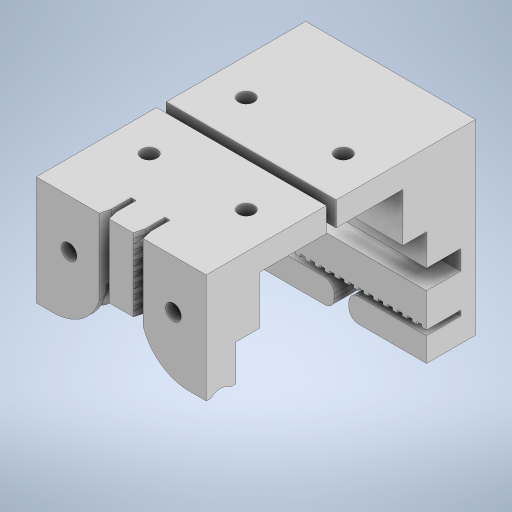
# Autodesk Inventor part: carriage
Saved by Autodesk Inventor 2023.1 (Build 271208000, 208)
## iProperties
Created: 2022-11-02
Part Number: carriage
Material: Generic
Document SubType Name: Modeling
Designer: nicol
Density: 1 g/cm^3
Appearance: Default
Author: nicol
Autodesk Inventor part; units mm, degrees
ref_plane "YZ Plane" through (0, 0, 0) normal (1, 0, 0) x (0, 1, 0)
ref_plane "XZ Plane" through (0, 0, 0) normal (0, 1, 0) x (-1, 0, 0)
ref_plane "XY Plane" through (0, 0, 0) normal (0, 0, 1) x (1, 0, 0)
sketch "Sketch1" plane through (0, 0, 0) normal (0, 1, 0) x (-1, 0, 0)
  line L0 (0, 0) -> (35, 0)
  line L1 (35, 0) -> (35, -55.5)
  line L2 (35, -55.5) -> (0, -55.5)
  line L3 (0, -55.5) -> (0, 0)
  line L4 (27.5, -15.75) -> (7.5, -15.75) construction
  line L5 (7.5, -15.75) -> (7.5, -35.75) construction
  line L6 (7.5, -35.75) -> (27.5, -35.75) construction
  line L7 (27.5, -35.75) -> (27.5, -15.75) construction
  dimension "d0" = 20
  dimension "d1" = 20
  dimension "d2" = 15.75
  dimension "d3" = 19.75
  dimension "d4" = 35
  dimension "d5" = 7.5
  dimension "d6" = 7.5
  constraints: 16 end point, 4 parallel, 2 horizontal, 2 perpendicular
  measures "d0" distance of L6.end L5.end
  measures "d1" distance of L5.end L4.end
  measures "d2" distance between parallel lines of L0 L4
  measures "d3" distance between parallel lines of L2 L6
  measures "d4" distance of L0.start L0.end
  measures "d5" distance between parallel lines of L1 L7
  measures "d6" distance between parallel lines of L3 L5
extrude "Extrusion1" add sketch "Sketch1" against normal blind 5
hole "Hole1" at (-27.5, 0, -15.75) at (-7.5, 0, -15.75) at (-27.5, 0, -35.75) at (-7.5, 0, -35.75) direction (0, -1, 0) diameter 3.2 end through all
sketch "Sketch2" plane through (0, -5, 0) normal (0, -1, 0) x (1, 0, 0)
  circle A0 centre (-27.5, -35.75) radius 1.6 projected
  circle A1 centre (-27.5, -15.75) radius 1.6 projected
  circle A2 centre (-7.5, -15.75) radius 1.6 projected
  circle A3 centre (-7.5, -35.75) radius 1.6 projected
  line L0 (-35, -55.5) -> (0, -55.5) projected
  line L1 (0, -55.5) -> (0, 0) projected
  line L2 (0, 0) -> (-35, 0) projected
  line L3 (-35, 0) -> (-35, -55.5) projected
  line L4 (0, -40.5) -> (-35, -40.5)
  line L5 (-35, -55.5) -> (-35, 0) projected
  line L6 (-35, -11) -> (0, -11)
  line L7 (0, 0) -> (0, -55.5) projected
  point P0 (0, -11)
  dimension "d16" = 11
  dimension "d17" = 15
  constraints: 4 end point, 4 point on line, 1 horizontal, 1 parallel
  measures "d16" distance between parallel lines of L2 L6
  measures "d17" distance between parallel lines of L0 L4
extrude "Extrusion2" add sketch "Sketch2" along normal blind 17.5 contours L3 L4 L1 L0 | L3 L2 L1 L6
sketch "Sketch4" plane through (-35, 0, 0) normal (0, 0, 1) x (1, 0, 0)
  line L0 (0, -22.5) -> (3.5, -22.5)
  line L1 (0, 0) -> (35, 0) projected
  line L2 (0, 0) -> (0, -22.5) projected
  line L3 (35, -22.5) -> (0, -22.5) projected
  line L4 (35, 0) -> (35, -22.5) projected
  line L5 (0, -22.5) -> (0, -26) construction
  line L6 (0, -5) -> (0, -22.5) construction
  circle A0 centre (-97.8915, -18) radius 4.5 construction
  line L7 (15, 0) -> (20, 0)
  line L8 (20, 0) -> (20, -15)
  line L9 (20, -15) -> (15, -15)
  line L10 (15, -15) -> (15, 0)
  line L11 (13.5, 0) -> (13.5, -12.5)
  arc A1 (3.5, -22.5) -> (13.5, -12.5) centre (3.5, -12.5) ccw
  line L12 (15, 0) -> (14.5, 0)
  line L13 (14.5, 0) -> (14.5, -1)
  line L14 (14.5, -1) -> (15, -1)
  line L15 (15, -1) -> (15, 0)
  line L16 (20, 0) -> (20.5, 0)
  line L17 (20.5, 0) -> (20.5, -1)
  line L18 (20.5, -1) -> (20, -1)
  line L19 (20, -1) -> (20, 0)
  line L20 (21.5, 0) -> (21.5, -12.5)
  line L21 (35, 0) -> (35, -22.5) projected
  line L22 (35, -22.5) -> (31.5, -22.5)
  arc A2 (21.5, -12.5) -> (31.5, -22.5) centre (31.5, -12.5) ccw
  line L23 (15, 0) -> (14.5, -0.5) construction
  line L24 (15, -1) -> (14.5, -0.5) construction
  line L25 (20, 0) -> (20.5, -0.5) construction
  line L26 (20, -1) -> (20.5, -0.5) construction
  line L27 (20, -3) -> (20.5, -2.5) construction
  line L28 (20, -3) -> (20, -2)
  line L29 (20, -2) -> (20.5, -2)
  line L30 (20, -2) -> (20.5, -2.5) construction
  line L31 (20.5, -3) -> (20, -3)
  line L32 (20.5, -2) -> (20.5, -3)
  line L33 (15, -2) -> (14.5, -2.5) construction
  line L34 (15, -3) -> (15, -2)
  line L35 (14.5, -3) -> (15, -3)
  line L36 (14.5, -2) -> (14.5, -3)
  line L37 (15, -2) -> (14.5, -2)
  line L38 (15, -3) -> (14.5, -2.5) construction
  line L39 (20, -5) -> (20.5, -4.5) construction
  line L40 (20, -5) -> (20, -4)
  line L41 (20, -4) -> (20.5, -4)
  line L42 (20, -4) -> (20.5, -4.5) construction
  line L43 (20.5, -5) -> (20, -5)
  line L44 (20.5, -4) -> (20.5, -5)
  line L45 (15, -4) -> (14.5, -4.5) construction
  line L46 (15, -5) -> (15, -4)
  line L47 (14.5, -5) -> (15, -5)
  line L48 (14.5, -4) -> (14.5, -5)
  line L49 (15, -4) -> (14.5, -4)
  line L50 (15, -5) -> (14.5, -4.5) construction
  line L51 (20, -7) -> (20.5, -6.5) construction
  line L52 (20, -7) -> (20, -6)
  line L53 (20, -6) -> (20.5, -6)
  line L54 (20, -6) -> (20.5, -6.5) construction
  line L55 (20.5, -7) -> (20, -7)
  line L56 (20.5, -6) -> (20.5, -7)
  line L57 (15, -6) -> (14.5, -6.5) construction
  line L58 (15, -7) -> (15, -6)
  line L59 (14.5, -7) -> (15, -7)
  line L60 (14.5, -6) -> (14.5, -7)
  line L61 (15, -6) -> (14.5, -6)
  line L62 (15, -7) -> (14.5, -6.5) construction
  line L63 (20, -9) -> (20.5, -8.5) construction
  line L64 (20, -9) -> (20, -8)
  line L65 (20, -8) -> (20.5, -8)
  line L66 (20, -8) -> (20.5, -8.5) construction
  line L67 (20.5, -9) -> (20, -9)
  line L68 (20.5, -8) -> (20.5, -9)
  line L69 (15, -8) -> (14.5, -8.5) construction
  line L70 (15, -9) -> (15, -8)
  line L71 (14.5, -9) -> (15, -9)
  line L72 (14.5, -8) -> (14.5, -9)
  line L73 (15, -8) -> (14.5, -8)
  line L74 (15, -9) -> (14.5, -8.5) construction
  line L75 (20, -11) -> (20.5, -10.5) construction
  line L76 (20, -11) -> (20, -10)
  line L77 (20, -10) -> (20.5, -10)
  line L78 (20, -10) -> (20.5, -10.5) construction
  line L79 (20.5, -11) -> (20, -11)
  line L80 (20.5, -10) -> (20.5, -11)
  line L81 (15, -10) -> (14.5, -10.5) construction
  line L82 (15, -11) -> (15, -10)
  line L83 (14.5, -11) -> (15, -11)
  line L84 (14.5, -10) -> (14.5, -11)
  line L85 (15, -10) -> (14.5, -10)
  line L86 (15, -11) -> (14.5, -10.5) construction
  line L87 (20, -13) -> (20.5, -12.5) construction
  line L88 (20, -13) -> (20, -12)
  line L89 (20, -12) -> (20.5, -12)
  line L90 (20, -12) -> (20.5, -12.5) construction
  line L91 (20.5, -13) -> (20, -13)
  line L92 (20.5, -12) -> (20.5, -13)
  line L93 (15, -12) -> (14.5, -12.5) construction
  line L94 (15, -13) -> (15, -12)
  line L95 (14.5, -13) -> (15, -13)
  line L96 (14.5, -12) -> (14.5, -13)
  line L97 (15, -12) -> (14.5, -12)
  line L98 (15, -13) -> (14.5, -12.5) construction
  line L99 (20, -15) -> (20.5, -14.5) construction
  line L100 (20, -15) -> (20, -14)
  line L101 (20, -14) -> (20.5, -14)
  line L102 (20, -14) -> (20.5, -14.5) construction
  line L103 (20.5, -15) -> (20, -15)
  line L104 (20.5, -14) -> (20.5, -15)
  line L105 (15, -14) -> (14.5, -14.5) construction
  line L106 (15, -15) -> (15, -14)
  line L107 (14.5, -15) -> (15, -15)
  line L108 (14.5, -14) -> (14.5, -15)
  line L109 (15, -14) -> (14.5, -14)
  line L110 (15, -15) -> (14.5, -14.5) construction
  point P0 (0, -24.25)
  point P1 (17.5, 0)
  point P2 (14.5, 0)
  point P3 (3.5, -22.5)
  point P4 (31.5, -22.5)
  dimension "d48" = 5
  dimension "d49" = 1.5
  dimension "d50" = 0.5
  dimension "d51" = 1
  dimension "d59" = 10
  dimension "d60" = 0.5
  dimension "d61" = 1
  dimension "d88" = 15
  dimension "d210" = 2
  constraints: 210 end point, 6 parallel, 6 point on line, 5 midpoint, 5 tangent, 4 horizontal, 4 point on circle, 3 perpendicular, 3 vertical, 2 centre point, 2 collinear, 2 equal length, 154 other
  measures "d48" distance of L8.end L9.end
  measures "d49" distance between parallel lines of L10 L11
  measures "d50" distance of L13.end L14.end
  measures "d51" distance of L12.end L13.end
  measures "d59" radius of A1
  measures "d60" distance of L17.end L18.end
  measures "d61" distance of L16.end L17.end
  measures "d88" distance between parallel lines of L1 L9
  measures "d210" distance of L18.end L27.start
extrude "Extrusion5" cut sketch "Sketch4" against normal blind 6 contours A1 L11 L1 L13 L14 L10 L37 L36 L35 L49 L48 L47 L61 L60 L59 L73 L72 L71 L85 L84 L83 L97 L96 L95 L109 L108 L107 L9 L103 L104 L101 L8 L91 L92 L89 L79 L80 L77 L67 L68 L65 L55 L56 L53 L43 L44 L41 L31 L32 L29 L18 L17 L20 A2 L3
sketch "Sketch5" plane through (-35, 0, -6) normal (0, 0, 1) x (1, 0, 0)
  line L0 (15, -9) -> (15, -10) projected
  line L1 (13.5, 0) -> (14.5, 0) projected
  line L2 (31.5, -22.5) -> (3.5, -22.5) projected
  arc A0 (21.5, -12.5) -> (31.5, -22.5) centre (31.5, -12.5) ccw projected
  line L3 (21.5, 0) -> (21.5, -12.5) projected
  line L4 (20.5, 0) -> (21.5, 0) projected
  line L5 (20, -2) -> (20, -1) projected
  line L6 (14.5, -15) -> (20.5, -15) projected
  line L7 (21.8175, -15) -> (12.9325, -15)
  line L8 (14.5, -15) -> (20.5, -15) projected
  line L9 (15, -14) -> (14.5, -14) projected
  line L10 (15, -13) -> (15, -14) projected
  line L11 (14.5, -13) -> (15, -13) projected
  line L12 (14.5, -12) -> (14.5, -13) projected
  line L13 (15, -12) -> (14.5, -12) projected
  line L14 (15, -11) -> (15, -12) projected
  line L15 (14.5, -11) -> (15, -11) projected
  line L16 (14.5, -10) -> (14.5, -11) projected
  line L17 (15, -10) -> (14.5, -10) projected
  line L18 (14.5, -9) -> (15, -9) projected
  line L19 (14.5, -8) -> (14.5, -9) projected
  line L20 (15, -8) -> (14.5, -8) projected
  line L21 (15, -7) -> (15, -8) projected
  line L22 (14.5, -7) -> (15, -7) projected
  line L23 (14.5, -6) -> (14.5, -7) projected
  line L24 (15, -6) -> (14.5, -6) projected
  line L25 (15, -5) -> (15, -6) projected
  line L26 (14.5, -5) -> (15, -5) projected
  line L27 (14.5, -4) -> (14.5, -5) projected
  line L28 (15, -4) -> (14.5, -4) projected
  line L29 (15, -3) -> (15, -4) projected
  line L30 (14.5, -3) -> (15, -3) projected
  line L31 (14.5, -2) -> (14.5, -3) projected
  line L32 (15, -2) -> (14.5, -2) projected
  line L33 (15, -1) -> (15, -2) projected
  line L34 (14.5, -1) -> (15, -1) projected
  line L35 (14.5, 0) -> (14.5, -1) projected
  line L36 (13.5, -12.5) -> (13.5, 0) projected
  arc A1 (3.5, -22.5) -> (13.5, -12.5) centre (3.5, -12.5) ccw projected
  line L37 (20.5, -1) -> (20.5, 0) projected
  line L38 (20, -1) -> (20.5, -1) projected
  line L39 (20.5, -2) -> (20, -2) projected
  line L40 (20.5, -3) -> (20.5, -2) projected
  line L41 (20, -3) -> (20.5, -3) projected
  line L42 (20, -4) -> (20, -3) projected
  line L43 (20.5, -4) -> (20, -4) projected
  line L44 (20.5, -5) -> (20.5, -4) projected
  line L45 (20, -5) -> (20.5, -5) projected
  line L46 (20, -6) -> (20, -5) projected
  line L47 (20.5, -6) -> (20, -6) projected
  line L48 (20.5, -7) -> (20.5, -6) projected
  line L49 (20, -7) -> (20.5, -7) projected
  line L50 (20, -8) -> (20, -7) projected
  line L51 (20.5, -8) -> (20, -8) projected
  line L52 (20.5, -9) -> (20.5, -8) projected
  line L53 (20, -9) -> (20.5, -9) projected
  line L54 (20, -10) -> (20, -9) projected
  line L55 (20.5, -10) -> (20, -10) projected
  line L56 (20.5, -11) -> (20.5, -10) projected
  line L57 (20, -11) -> (20.5, -11) projected
  line L58 (20, -12) -> (20, -11) projected
  line L59 (20.5, -12) -> (20, -12) projected
  line L60 (20.5, -13) -> (20.5, -12) projected
  line L61 (20, -13) -> (20.5, -13) projected
  line L62 (20, -14) -> (20, -13) projected
  line L63 (20.5, -14) -> (20, -14) projected
  line L64 (20.5, -15) -> (20.5, -14) projected
  line L65 (14.5, -14) -> (14.5, -15) projected
  point P0 (35, 0)
  point P1 (15, -15)
  point P2 (20, -15)
  point P3 (15, -15)
  point P4 (20, -15)
  point P5 (13.1825, -15)
  constraints: 2 end point, 1 collinear, 1 point on circle
extrude "Extrusion6" cut sketch "Sketch5" against normal blind 7 contours L6 L7 A0 L2 A1
sketch "Sketch6" plane through (-35, 0, -55.5) normal (-1, 0, 0) x (0, 0, 1)
  line L0 (0, 0) -> (55.5, 0) projected
  line L1 (0, 0) -> (0, -22.5) projected
  line L2 (15, -22.5) -> (0, -22.5) projected
  line L3 (15, -5) -> (15, -22.5) projected
  line L4 (44.5, -5) -> (15, -5) projected
  line L5 (44.5, -22.5) -> (55.5, -22.5) projected
  arc A0 (54.5, -22.5) -> (50.5, -22.5) centre (52.5, -24.7361) ccw
  line L6 (44.5, -5) -> (44.5, -22.5) projected
  line L7 (55.5, -22.5) -> (44.5, -22.5) projected
  line L8 (49.5, -12.5) -> (49.5, -15) projected
  line L9 (55.5, 0) -> (55.5, -22.5) projected
  line L10 (49.5, -15) -> (49.5, -12.5) projected
  line L11 (49.5, -14) -> (49.5, -15) projected
  line L12 (49.5, -13) -> (49.5, -14) projected
  line L13 (49.5, -12) -> (49.5, -13) projected
  line L14 (49.5, -11) -> (49.5, -12) projected
  line L15 (49.5, -10) -> (49.5, -11) projected
  line L16 (49.5, -9) -> (49.5, -10) projected
  line L17 (49.5, -8) -> (49.5, -9) projected
  line L18 (49.5, -7) -> (49.5, -8) projected
  line L19 (49.5, -6) -> (49.5, -7) projected
  line L20 (49.5, -5) -> (49.5, -6) projected
  line L21 (49.5, -4) -> (49.5, -5) projected
  line L22 (49.5, -3) -> (49.5, -4) projected
  line L23 (49.5, -2) -> (49.5, -3) projected
  line L24 (49.5, -1) -> (49.5, -2) projected
  line L25 (49.5, 0) -> (49.5, -1) projected
  line L26 (49.5, -12.5) -> (49.5, 0) projected
  line L27 (49.5, 0) -> (49.5, -12.5) projected
  line L28 (49.5, -1) -> (49.5, 0) projected
  line L29 (49.5, -2) -> (49.5, -1) projected
  line L30 (49.5, -3) -> (49.5, -2) projected
  line L31 (49.5, -4) -> (49.5, -3) projected
  line L32 (49.5, -5) -> (49.5, -4) projected
  line L33 (49.5, -6) -> (49.5, -5) projected
  line L34 (49.5, -7) -> (49.5, -6) projected
  line L35 (49.5, -8) -> (49.5, -7) projected
  line L36 (49.5, -9) -> (49.5, -8) projected
  line L37 (49.5, -10) -> (49.5, -9) projected
  line L38 (49.5, -11) -> (49.5, -10) projected
  line L39 (49.5, -12) -> (49.5, -11) projected
  line L40 (49.5, -13) -> (49.5, -12) projected
  line L41 (49.5, -14) -> (49.5, -13) projected
  line L42 (49.5, -15) -> (49.5, -14) projected
  point P0 (49.5, -22.5)
  dimension "d73" = 1
  dimension "d74" = 1
  dimension "d75" = 3
  constraints: 2 point on circle, 2 point on line, 1 centre point
  measures "d73" distance of L5.end A0.start
  measures "d74" horizontal distance of L10.start A0.end
  measures "d75" radius of A0
sketch3d "3D Sketch1"
  line L0 (-35, -22.5, 0) -> (-31.5, -22.5, 0)
  arc A0 (-31.5, -22.5, 0) -> (-21.5, -12.5, 0) centre (-31.5, -12.5, 0) ccw
sweep "Sweep1" cut profiles "Sketch6" path "3D Sketch1" contours L5 A0
chamfer "Chamfer1" distance 0.75 angle 45 1 edges at (-22.2639, -12.5, -3)
ref_plane "Work Plane3" through (-17.5, 0, 0) normal (1, 0, 0) x (0, 0, -1)
mirror "Mirror2" about plane through (-17.5, 0, 0) normal (1, 0, 0) of "Sweep1", "Chamfer1"
sketch "Sketch7" plane through (0, -5, -11) normal (0, 0, -1) x (-1, 0, 0)
  line L0 (35, -17.5) -> (31.5, -17.5) projected
  line L1 (35, 0) -> (35, -17.5) projected
  line L2 (0, 0) -> (35, 0) projected
  line L3 (0, 0) -> (0, -17.5) projected
  arc A0 (3.5, -17.5) -> (13.1825, -10) centre (3.5, -7.5) ccw projected
  line L4 (0, 0) -> (0, -17.5) projected
  line L5 (0, -10) -> (13.1825, -10)
  line L6 (21.8175, -10) -> (35, -10)
  line L7 (35, 0) -> (35, -17.5) projected
  arc A1 (21.8175, -10) -> (31.5, -17.5) centre (31.5, -7.5) ccw projected
  line L8 (3.5, -17.5) -> (0, -17.5) projected
  line L9 (13.1825, -10) -> (21.8175, -10) projected
  point P0 (0, 5)
  constraints: 4 end point, 3 point on line, 1 perpendicular
extrude "Extrusion7" cut sketch "Sketch7" against normal blind 4.9 contours L0 A1 L6 L1 | A0 L8 L3 L5
sketch "Sketch9" plane through (0, -22.5, 0) normal (0, -1, 0) x (1, 0, 0)
  line L0 (0, -55.5) -> (0, -40.5) projected
  line L1 (0, -40.5) -> (-35, -40.5) projected
  line L2 (-35, -40.5) -> (-35, -55.5) projected
  line L3 (-35, -55.5) -> (0, -55.5) projected
  point P0 (0, 0)
extrude "Extrusion8" add sketch "Sketch9" along normal blind 16
sketch "Sketch8" plane through (0, 0, -40.5) normal (0, 0, -1) x (-1, 0, 0)
  line L0 (0, -33.5) -> (14, -33.5)
  line L1 (21, -33.5) -> (35, -33.5)
  line L2 (19, -35.5) -> (19, -36.5)
  line L3 (16, -35.5) -> (16, -36.5)
  arc A0 (16, -35.5) -> (14, -33.5) centre (14, -35.5) ccw
  arc A1 (21, -33.5) -> (19, -35.5) centre (21, -35.5) ccw
  arc A2 (19, -36.5) -> (21, -38.5) centre (21, -36.5) ccw
  arc A3 (14, -38.5) -> (16, -36.5) centre (14, -36.5) ccw
  line L4 (35, -38.5) -> (0, -38.5) projected
  line L5 (0, 0) -> (35, 0) projected
  line L6 (0, 0) -> (0, -38.5) projected
  line L7 (35, -38.5) -> (0, -38.5) projected
  line L8 (35, 0) -> (35, -38.5) projected
  line L9 (0, -21.5) -> (35, -21.5)
  line L10 (35, -21.5) -> (35, -25.5)
  line L11 (35, -25.5) -> (0, -25.5)
  line L12 (0, -25.5) -> (0, -21.5)
  line L13 (35, 0) -> (35, -38.5) projected
  line L14 (0, 0) -> (0, -38.5) projected
  line L15 (0, -25.5) -> (35, -25.5)
  line L16 (35, -25.5) -> (35, -32)
  line L17 (35, -32) -> (0, -32)
  line L18 (0, -32) -> (0, -25.5)
  line L19 (35, -15) -> (0, -15)
  line L20 (0, -5) -> (0, -38.5) projected
  line L21 (35, -5) -> (0, -5) projected
  line L22 (0, -32) -> (1, -32)
  line L23 (1, -32) -> (1, -32.5)
  line L24 (1, -32.5) -> (0, -32.5)
  line L25 (0, -32.5) -> (0, -32)
  line L26 (2, -32) -> (3, -32)
  line L27 (2, -32.5) -> (2, -32)
  line L28 (3, -32) -> (3, -32.5)
  line L29 (3, -32.5) -> (2, -32.5)
  line L30 (4, -32) -> (5, -32)
  line L31 (4, -32.5) -> (4, -32)
  line L32 (5, -32) -> (5, -32.5)
  line L33 (5, -32.5) -> (4, -32.5)
  line L34 (6, -32) -> (7, -32)
  line L35 (6, -32.5) -> (6, -32)
  line L36 (7, -32) -> (7, -32.5)
  line L37 (7, -32.5) -> (6, -32.5)
  line L38 (8, -32) -> (9, -32)
  line L39 (8, -32.5) -> (8, -32)
  line L40 (9, -32) -> (9, -32.5)
  line L41 (9, -32.5) -> (8, -32.5)
  line L42 (10, -32) -> (11, -32)
  line L43 (10, -32.5) -> (10, -32)
  line L44 (11, -32) -> (11, -32.5)
  line L45 (11, -32.5) -> (10, -32.5)
  line L46 (12, -32) -> (13, -32)
  line L47 (12, -32.5) -> (12, -32)
  line L48 (13, -32) -> (13, -32.5)
  line L49 (13, -32.5) -> (12, -32.5)
  line L50 (14, -32) -> (15, -32)
  line L51 (14, -32.5) -> (14, -32)
  line L52 (15, -32) -> (15, -32.5)
  line L53 (15, -32.5) -> (14, -32.5)
  line L54 (16, -32) -> (17, -32)
  line L55 (16, -32.5) -> (16, -32)
  line L56 (17, -32) -> (17, -32.5)
  line L57 (17, -32.5) -> (16, -32.5)
  line L58 (18, -32) -> (19, -32)
  line L59 (18, -32.5) -> (18, -32)
  line L60 (19, -32) -> (19, -32.5)
  line L61 (19, -32.5) -> (18, -32.5)
  line L62 (20, -32) -> (21, -32)
  line L63 (20, -32.5) -> (20, -32)
  line L64 (21, -32) -> (21, -32.5)
  line L65 (21, -32.5) -> (20, -32.5)
  line L66 (22, -32) -> (23, -32)
  line L67 (22, -32.5) -> (22, -32)
  line L68 (23, -32) -> (23, -32.5)
  line L69 (23, -32.5) -> (22, -32.5)
  line L70 (24, -32) -> (25, -32)
  line L71 (24, -32.5) -> (24, -32)
  line L72 (25, -32) -> (25, -32.5)
  line L73 (25, -32.5) -> (24, -32.5)
  line L74 (26, -32) -> (27, -32)
  line L75 (26, -32.5) -> (26, -32)
  line L76 (27, -32) -> (27, -32.5)
  line L77 (27, -32.5) -> (26, -32.5)
  line L78 (28, -32) -> (29, -32)
  line L79 (28, -32.5) -> (28, -32)
  line L80 (29, -32) -> (29, -32.5)
  line L81 (29, -32.5) -> (28, -32.5)
  line L82 (30, -32) -> (31, -32)
  line L83 (30, -32.5) -> (30, -32)
  line L84 (31, -32) -> (31, -32.5)
  line L85 (31, -32.5) -> (30, -32.5)
  line L86 (32, -32) -> (33, -32)
  line L87 (32, -32.5) -> (32, -32)
  line L88 (33, -32) -> (33, -32.5)
  line L89 (33, -32.5) -> (32, -32.5)
  line L90 (34, -32) -> (35, -32)
  line L91 (34, -32.5) -> (34, -32)
  line L92 (35, -32) -> (35, -32.5)
  line L93 (35, -32.5) -> (34, -32.5)
  point P0 (0, -32)
  point P1 (0, -21.5)
  point P2 (35, -32.5)
  point P3 (15, -32)
  point P4 (14, -32)
  point P5 (13, -32)
  point P6 (12, -32)
  point P7 (11, -32)
  point P8 (10, -32)
  point P9 (8, -32)
  point P10 (7, -32)
  point P11 (6, -32)
  point P12 (4, -32)
  point P13 (3, -32)
  point P14 (2, -32)
  point P15 (1, -32)
  point P16 (0, -32.5)
  dimension "d167" = 17
  dimension "d168" = 4
  dimension "d169" = 2
  dimension "d173" = 3
  dimension "d174" = 5
  dimension "d175" = 1.5
  dimension "d176" = 10
  dimension "d199" = 1
  dimension "d200" = 0.5
  dimension "d203" = 2
  constraints: 168 end point, 68 horizontal alignment, 39 parallel, 36 collinear, 8 point on circle, 8 tangent, 7 point on line, 6 horizontal, 4 centre point, 4 perpendicular, 3 equal radius, 2 equal length, 2 vertical, 3 other
  measures "d167" distance between parallel lines of L4 L9
  measures "d168" distance between parallel lines of L9 L11
  measures "d169" radius of A0
  measures "d173" distance between parallel lines of L2 L3
  measures "d174" distance between parallel lines of L7 L0
  measures "d176" distance between parallel lines of L21 L19
  measures "d199" distance of L23.end L24.end
  measures "d200" distance of L22.end L23.end
  measures "d203" distance of L18.start L26.start
extrude "Extrusion9" cut sketch "Sketch8" along normal blind 4.9 from surface at 0 contours L6 L24 L23 L17 L27 L29 L28 L31 L33 L32 L35 L37 L36 L39 L41 L40 L43 L45 L44 L47 L49 L48 L51 L53 L52 L55 L57 L56 L59 L61 L60 L63 L65 L64 L67 L69 L68 L71 L73 L72 L75 L77 L76 L79 L81 L80 L83 L85 L84 L87 L89 L88 L91 L93 L8 L1 A1 L2 A2 L4 A3 L3 A0 L0 | L0 A0 L3 A3 L4 L6 | L6 L17 L23 L24 | L6 L11 L8 L17 | L6 L9 L8 L11 | A2 L2 A1 L1 L8 L4 | L6 L19 L8 L9 | L17 L28 L29 L27 | L8 L93 L91 L17 | L17 L32 L33 L31 | L88 L89 L87 L17 | L17 L36 L37 L35 | L84 L85 L83 L17 | L17 L40 L41 L39 | L80 L81 L79 L17 | L17 L44 L45 L43 | L76 L77 L75 L17 | L17 L48 L49 L47 | L72 L73 L71 L17 | L17 L52 L53 L51 | L68 L69 L67 L17 | L17 L56 L57 L55 | L64 L65 L63 L17 | L17 L60 L61 L59
extrude "Extrusion17" cut sketch "Sketch8" along normal blind 7 from surface at 4.9 contours L6 L24 L23 L17 L27 L29 L28 L31 L33 L32 L35 L37 L36 L39 L41 L40 L43 L45 L44 L47 L49 L48 L51 L53 L52 L55 L57 L56 L59 L61 L60 L63 L65 L64 L67 L69 L68 L71 L73 L72 L75 L77 L76 L79 L81 L80 L83 L85 L84 L87 L89 L88 L91 L93 L8 L1 A1 L2 A2 L4 A3 L3 A0 L0 | L6 L9 L8 L11
sketch "Sketch14" plane through (-35, -22.5, 0) normal (0, 0, 1) x (1, 0, 0)
  line L0 (0, 17.5) -> (0, 7.5) projected
  line L1 (35, 17.5) -> (35, 7.5) projected
  line L2 (9.55, 10.8834) -> (6.75, 9.2668)
  line L3 (6.75, 9.2668) -> (3.95, 10.8834)
  line L4 (3.95, 10.8834) -> (3.95, 14.1166)
  line L5 (3.95, 14.1166) -> (6.75, 15.7332)
  line L6 (6.75, 15.7332) -> (9.55, 14.1166)
  line L7 (9.55, 14.1166) -> (9.55, 10.8834)
  line L8 (28.25, 9.2668) -> (25.45, 10.8834)
  line L9 (25.45, 10.8834) -> (25.45, 14.1166)
  line L10 (25.45, 14.1166) -> (28.25, 15.7332)
  line L11 (28.25, 15.7332) -> (31.05, 14.1166)
  line L12 (31.05, 14.1166) -> (31.05, 10.8834)
  line L13 (31.05, 10.8834) -> (28.25, 9.2668)
  line L14 (21.5, 22.5) -> (21.5, 10) projected
  line L15 (0, 17.5) -> (35, 17.5) projected
  line L16 (21.5, 17.5) -> (35, 17.5)
  line L17 (13.5, 10) -> (13.5, 22.5) projected
  line L18 (13.5, 17.5) -> (0, 17.5)
  line L19 (35, 17.5) -> (0, 17.5) projected
  line L20 (35, 7.5) -> (0, 7.5) projected
  point P0 (35, 22.5)
  point P1 (6.75, 12.5)
  point P2 (28.25, 12.5)
  point P3 (0, 12.5)
  point P4 (35, 12.5)
  point P5 (6.75, 17.5)
  point P6 (28.25, 17.5)
  dimension "d120" = 5.6
  constraints: 28 end point, 4 midpoint, 3 point on line, 2 horizontal alignment, 2 vertical, 2 vertical alignment, 1 horizontal, 1 parallel, 26 other
  measures "d120" distance between parallel lines of L7 L4
extrude "Extrusion12" cut sketch "Sketch14" along normal blind 8 from surface at -11 contours L2 L3 L4 L5 L6 L7 | L8 L9 L10 L11 L12 L13
hole "Hole4" at (-28.25, -10, 0) at (-6.75, -10, 0) direction (0, 0, -1) diameter 3.2 depth 11 tip angle 118
sketch "Sketch22" plane through (0, 0, 0) normal (0, 1, 0) x (1, 0, 0)
  line L0 (16.0256, 24.75) -> (-78.6573, 24.75)
  line L1 (-78.6573, 24.75) -> (-78.6573, 26.75)
  line L2 (-78.6573, 26.75) -> (16.0256, 26.75)
  line L3 (16.0256, 26.75) -> (16.0256, 24.75)
  circle A0 centre (-7.5, 15.75) radius 1.6 projected
  circle A1 centre (-7.5, 35.75) radius 1.6 projected
  line L4 (-7.5, 15.75) -> (-7.5, 35.75) construction
  point P0 (0, 0)
  point P1 (-31.3158, 24.75)
  point P2 (-7.5, 25.75)
  point P3 (16.0256, 25.75)
  dimension "d195" = 2
  constraints: 10 end point, 3 midpoint, 2 parallel, 1 horizontal, 1 horizontal alignment, 1 perpendicular, 1 vertical
  measures "d195" distance from line of point (-31.316, 24.75) L2
extrude "Extrusion20" cut sketch "Sketch22" against normal through all contours L0 L1 L2 L3
sketch "Sketch23" plane through (0, 0, 0) normal (0, 1, 0) x (1, 0, 0)
  line L0 (0, 24.75) -> (-35, 24.75) projected
  line L1 (-35, 24.75) -> (-35, 0) projected
  line L2 (-35, 0) -> (-21.5, 0) projected
  line L3 (-21.5, 0) -> (-21.5, 6) projected
  line L4 (-21.5, 6) -> (-20.5, 6) projected
  line L5 (-20.5, 6) -> (-20.5, 0) projected
  line L6 (-20.5, 0) -> (-14.5, 0) projected
  line L7 (-14.5, 0) -> (-14.5, 6) projected
  line L8 (-14.5, 6) -> (-13.5, 6) projected
  line L9 (-13.5, 6) -> (-13.5, 0) projected
  line L10 (-13.5, 0) -> (0, 0) projected
  line L11 (0, 0) -> (0, 24.75) projected
  circle A0 centre (-27.5, 15.75) radius 1.6 projected
  circle A1 centre (-7.5, 15.75) radius 1.6 projected
  line L12 (-14.5, 0) -> (-14.5, 6) projected
  line L13 (-14.5, 2) -> (-15, 0)
  line L14 (-20.5, 0) -> (-14.5, 0) projected
  line L15 (-13.5, 6) -> (-13.5, 0) projected
  line L16 (-13.5, 2) -> (-13, 0)
  line L17 (-20.5, 0) -> (-20.5, 6) projected
  line L18 (-20.5, 2) -> (-20, 0)
  line L19 (-21.5, 0) -> (-21.5, 6) projected
  line L20 (-21.5, 2) -> (-22, 0)
  dimension "d215" = 4
  dimension "d216" = 4
  dimension "d217" = 4
  dimension "d218" = 4
  dimension "d219" = 2
  dimension "d220" = 2
  dimension "d221" = 2
  dimension "d222" = 2
  dimension "d223" = 0.5
  constraints: 8 end point, 8 point on line, 3 equal length
  measures "d215" distance from line of L20.start L4
  measures "d216" distance of L4.end L18.start
  measures "d217" distance of L7.end L13.start
  measures "d218" distance of L8.end L16.start
  measures "d219" distance of L9.end L16.start
  measures "d220" distance of L6.end L13.start
  measures "d221" distance of L5.end L18.start
  measures "d222" distance of L2.end L20.start
  measures "d223" distance of L16.end L9.end
extrude "Extrusion21" cut sketch "Sketch23" against normal through all contours L10 L9 L16 | L20 L3 L2 | L7 L6 L13 | L18 L6 L5
equation "\"d5\" = d6"
body "Solid1"
